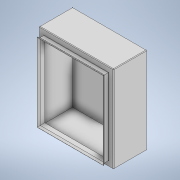
# Autodesk Inventor part: Box
Saved by Autodesk Inventor 2022 (Build 260153000, 153)
## iProperties
Created: 2024-10-27
Part Number: Box
Material: Ogólny
Document SubType Name: Modeling
Designer: NANOmatic
Density: 1 g/cm^3
Appearance: Domyślna
Author: NANOmatic
Autodesk Inventor part; units mm, degrees
ref_plane "YZ Plane" through (0, 0, 0) normal (1, 0, 0) x (0, 1, 0)
ref_plane "XZ Plane" through (0, 0, 0) normal (0, 1, 0) x (-1, 0, 0)
ref_plane "XY Plane" through (0, 0, 0) normal (0, 0, 1) x (1, 0, 0)
sketch "Szkic1" plane through (0, 0, 0) normal (0, 0, 1) x (1, 0, 0)
  line L0 (-150, 175) -> (150, 175)
  line L1 (150, 175) -> (150, -175)
  line L2 (150, -175) -> (-150, -175)
  line L3 (-150, -175) -> (-150, 175)
  line L4 (-150, 175) -> (150, -175) construction
  line L5 (150, 175) -> (-150, -175) construction
  point P0 (0, 0)
  dimension "d0" = 300
  dimension "d1" = 350
  constraints: 12 end point, 2 midpoint, 2 parallel, 1 horizontal, 1 perpendicular
  measures "d0" distance of L1.end L2.end
  measures "d1" distance of L0.end L1.end
extrude "Wyciągnięcie proste1" add sketch "Szkic1" along normal blind 135
sketch "Szkic2" plane through (0, 0, 0) normal (1, 0, 0) x (0, 1, 0)
  line L0 (-175, 135) -> (175, 135) projected
  line L1 (-157.1442, 138.8949) -> (-156.9942, 138.7449) construction
  line L2 (-156.3821, 159.375) -> (-152, 151.7849)
  line L3 (-152, 151.7849) -> (-152, 135)
  line L4 (-157.6812, 158.625) -> (-153.5, 151.383)
  line L5 (-153.5, 151.383) -> (-153.5, 135)
  line L6 (-152, 135) -> (-153.5, 135)
  line L7 (-156.3821, 159.375) -> (-157.6812, 158.625)
  point P0 (0, 0)
  dimension "d7" = 1.5
  dimension "d9" = 1.5
  dimension "d10" = 150
  dimension "d11" = 16.7849
  dimension "d12" = 8.7643
  dimension "d13" = 21.5
  constraints: 14 end point, 2 parallel, 1 collinear, 1 horizontal, 1 perpendicular, 1 vertical, 1 other
  measures "d7" distance of L3.end L5.end
  measures "d9" distance of L2.start L4.start
  measures "d10" angle of L4 L5
  measures "d11" distance of L2.end L3.end
  measures "d12" distance of L2.start L2.end
  measures "d13" distance from line of L5 L0.start
sketch "Szkic3" plane through (0, 0, 135) normal (0, 0, 1) x (1, 0, 0)
  line L0 (0, -152) -> (0, -153.5) projected
  line L1 (-129.2771, 152.75) -> (129.2771, 152.75)
  line L2 (129.2771, 152.75) -> (129.2771, -152.75)
  line L3 (129.2771, -152.75) -> (-129.2771, -152.75)
  line L4 (-129.2771, -152.75) -> (-129.2771, 152.75)
  line L5 (-129.2771, 152.75) -> (129.2771, -152.75) construction
  line L6 (129.2771, 152.75) -> (-129.2771, -152.75) construction
  line L7 (-150, -175) -> (-129.2771, -152.75) construction
  point P0 (0, 0)
  point P1 (0, -152.75)
  dimension "d14" = 30.4056
  constraints: 14 end point, 4 midpoint, 2 parallel, 1 horizontal, 1 perpendicular
  measures "d14" distance of L7.start L3.end
sweep "Przeciągnięcie1" add profiles "Szkic2" path "Szkic3" path curves L1 L4 L3 L2
shell "Skorupa1" thickness 1.5 removed faces 1 at (-42.8424, -50.6667, 135)
fillet "Zaokrąglenie1" radius 1 8 edges at (0, -153.5, 135) (-130.0271, 0, 135) (-130.0271, 0, 151.383) (0, -153.5, 151.383) (0, 153.5, 135) (0, 153.5, 151.383) (130.0271, 0, 135) (130.0271, 0, 151.383)
fillet "Zaokrąglenie1" radius 2.35 12 edges at (0, -175, 135) (150, 0, 135) (0, 175, 135) (-150, 0, 135) (0, -175, 0) (-150, 0, 0) (0, 175, 0) (150, 0, 0) (150, 175, 67.5) (150, -175, 67.5) (-150, -175, 67.5) (-150, 175, 67.5)
sketch "Szkic4" plane through (0, 0, 0) normal (0, 1, 0) x (-1, 0, 0)
  point P0 (0, 0)
  point P1 (139.675, 154.675)
  constraints: 1 other
equation "\"d9\" = d7"
equation "\"d14\" = 1.41421 * d13"
